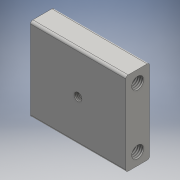
# Autodesk Inventor part: Profile_Middle_03
Saved by Autodesk Inventor 2016 (Build 200138000, 138)
## iProperties
Created: 2016-02-09
Part Number: Profile_Middle_03
Material: Generic
Document SubType Name: Modeling
Designer: nils
Density: 1 g/cm^3
Appearance: Default
Author: nils
Autodesk Inventor part; units mm, degrees
ref_plane "YZ Plane" through (0, 0, 0) normal (1, 0, 0) x (0, 1, 0)
ref_plane "XZ Plane" through (0, 0, 0) normal (0, 1, 0) x (-1, 0, 0)
sketch "Sketch1" plane through (0, 0, 0) normal (1, 0, 0) x (0, 1, 0)
  line L0 (-10, 35) -> (10, 35)
  line L1 (10, 35) -> (10, -35)
  line L2 (10, -35) -> (-10, -35)
  line L3 (-10, -35) -> (-10, 35)
  line L4 (-10, 35) -> (10, -35) construction
  line L5 (10, 35) -> (-10, -35) construction
  point P0 (0, 0)
  dimension "d0" = 20
  dimension "d1" = 70
  constraints: 12 end point, 2 midpoint, 2 parallel, 1 horizontal, 1 perpendicular
  measures "d0" distance of L1.end L2.end
  measures "d1" distance of L0.end L1.end
extrude "Extrusion1" add sketch "Sketch1" along normal blind 80
sketch "Sketch2" plane through (80, 0, 0) normal (1, 0, 0) x (0, 0, -1)
  line L0 (-35, 10) -> (-35, -10) projected
  line L1 (-35, 0) -> (35, 0)
  line L2 (35, -10) -> (35, 10) projected
  line L3 (35, 10) -> (-35, 10) projected
  line L4 (0, 10) -> (0, -10)
  line L5 (-35, -10) -> (35, -10) projected
  point P0 (0, 0)
  point P1 (-25, 0)
  point P2 (25, 0)
  dimension "d4" = 25
  constraints: 4 end point, 4 midpoint, 2 point on line, 1 symmetric about line
  measures "d4" distance from line of L4 point (-25, 0)
hole "Hole1" at (80, 0, 25) at (80, 0, -25) direction (-1, 0, 0) diameter 10.106 depth 24 tip angle 118 thread size "M12x1.75" class "6H" standard "ISO Metric profile"
ref_plane "Work Plane1" through (40, 0, 0) normal (1, 0, 0) x (0, 0, -1)
mirror "Mirror1" about plane through (40, 0, 0) normal (1, 0, 0) of "Hole1"
fillet "Fillet1" radius 2 4 edges at (40, 10, 35) (40, -10, 35) (40, -10, -35) (40, 10, -35)
sketch "Sketch3" plane through (0, 10, 33) normal (0, 1, 0) x (1, 0, 0)
  line L0 (80, 0) -> (80, 66) projected
  line L1 (80, 33) -> (0, 33)
  point P0 (40, 33)
  constraints: 2 end point, 2 midpoint, 1 horizontal
hole "Hole2" at (40, 10, 0) direction (0, -1, 0) diameter 6.647 end through all thread size "M8x1.25" class "6H" standard "ISO Metric profile"
body "Solid1"
